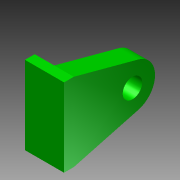
# Autodesk Inventor part: TabletMount-Base-Hinge
Saved by Autodesk Inventor 2012 (Build 160160000, 160)
## iProperties
Created: 2013-10-06
Part Number: TabletMount-Base-Hinge
Material: Default
Document SubType Name: Modeling
Designer: joe_000
Density: 1 g/cm^3
Author: joe_000
Autodesk Inventor part; units mm, degrees
ref_plane "YZ Plane" through (0, 0, 0) normal (1, 0, 0) x (0, 1, 0)
ref_plane "XZ Plane" through (0, 0, 0) normal (0, 1, 0) x (-1, 0, 0)
ref_plane "XY Plane" through (0, 0, 0) normal (0, 0, 1) x (1, 0, 0)
sketch "Sketch1" plane through (0, 0, 0) normal (1, 0, 0) x (0, 1, 0)
  line L0 (0, 0) -> (25.4, 0)
  line L1 (25.4, 0) -> (19.7868, -20.9489)
  line L2 (0, 0) -> (5.6132, -20.9489)
  line L3 (12.7, 0) -> (12.7, -162.0582)
  arc A0 (5.6132, -20.9489) -> (19.7868, -20.9489) centre (12.7, -19.05) ccw
  circle A1 centre (12.7, -19.05) radius 3.175
  dimension "d0" = 75
  dimension "d1" = 75
  dimension "d2" = 25.4
  dimension "d3" = 19.05
  dimension "d4" = 6.35
  constraints: 8 end point, 2 centre point, 2 point on circle, 1 coincident, 1 horizontal, 1 midpoint, 1 perpendicular, 1 point on line, 1 tangent
  measures "d0" angle of L1 L0
  measures "d1" angle of L2 L0
  measures "d2" distance of L0.start L0.end
  measures "d3" distance from line of L0 A0.centre
  measures "d4" diameter of A1
extrude "Extrusion1" add sketch "Sketch1" along normal blind 6.35 contours L0 L3 A1 A0 L2 | L0 L1 A0 L3 A1
sketch "Sketch2" plane through (0, 0, 0) normal (0, 0, 1) x (1, 0, 0)
  line L0 (6.35, 25.4) -> (-6.35, 25.4)
  line L1 (-6.35, 25.4) -> (-6.35, 0)
  line L2 (-6.35, 0) -> (6.35, 0)
  line L3 (6.35, 0) -> (6.35, 25.4)
  dimension "d7" = 12.7
  constraints: 8 end point, 2 parallel, 1 horizontal, 1 perpendicular
  measures "d7" distance of L0.start L0.end
extrude "Extrusion2" add sketch "Sketch2" along normal blind 3.175
equation "\"d1\" = d0"
body "Solid1"
